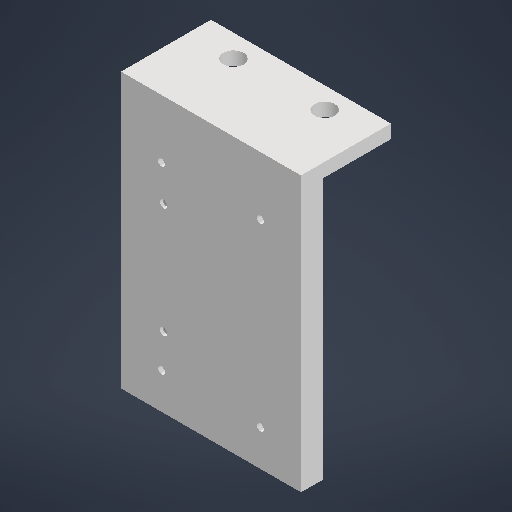
# Autodesk Inventor part: Support
Saved by Autodesk Inventor 2026.2 (Build 302298000, 298)
## iProperties
Created: 2025-11-07
Part Number: Support
Material: 일반
Document SubType Name: Modeling
Designer: alexi
Density: 1 g/cm^3
Appearance: 기본값
Author: alexi
Autodesk Inventor part; units mm, degrees
ref_plane "YZ Plane" through (0, 0, 0) normal (1, 0, 0) x (0, 1, 0)
ref_plane "XZ Plane" through (0, 0, 0) normal (0, 1, 0) x (-1, 0, 0)
ref_plane "XY Plane" through (0, 0, 0) normal (0, 0, 1) x (1, 0, 0)
ref_plane "작업 평면1" through (0, 0, 0) normal (0, 0, 1) x (1, 0, 0)
sketch "스케치1" plane through (0, 0, 0) normal (0, 0, 1) x (1, 0, 0)
  line L0 (15, -23) -> (15, 23) construction
  line L1 (15, 23) -> (-15, 23) construction
  line L2 (-15, 23) -> (-15, -23) construction
  line L3 (-15, -23) -> (15, -23) construction
  circle A0 centre (11, -20) radius 1.2 construction
  circle A1 centre (11, 20) radius 1.2 construction
  circle A2 centre (-11, -20) radius 1.2 construction
  circle A3 centre (-11, 20) radius 1.2 construction
  line L4 (20, 33) -> (-20, 33)
  line L5 (-20, 33) -> (-20, -28)
  line L6 (-20, -28) -> (20, -28)
  line L7 (20, -28) -> (20, 33)
  line L8 (-20, 30) -> (20, 30)
  line L9 (-15.525, 9.775) -> (15.475, 9.775)
  line L10 (15.475, 9.775) -> (15.475, -9.775)
  line L11 (15.475, -9.775) -> (-15.525, -9.775)
  line L12 (-15.525, -9.775) -> (-15.525, 9.775)
  circle A4 centre (-10.525, 12.275) radius 1.4
  circle A5 centre (-10.525, -12.275) radius 1.4
  point P0 (0, 0)
  dimension "d0" = 5
  dimension "d1" = 5
  dimension "d2" = 5
  dimension "d3" = 10
  dimension "d4" = 3
  dimension "d5" = 5
  dimension "d6" = 26
  dimension "d39" = 2.5
  dimension "d40" = 2.5
  constraints: 26 end point, 6 centre point, 4 horizontal, 4 parallel, 3 perpendicular, 2 point on line, 2 vertical, 17 other
  measures "d0" distance between parallel lines of L5 L2
  measures "d1" distance between parallel lines of L7 L0
  measures "d2" distance between parallel lines of L6 L3
  measures "d3" distance between parallel lines of L4 L1
  measures "d4" distance between parallel lines of L4 L8
  measures "d5" distance from line of L12 A4.centre
  measures "d6" distance from line of L10 A4.centre
  measures "d39" distance from line of L9 A4.centre
  measures "d40" distance from line of L11 A5.centre
extrude "돌출1" add sketch "스케치1" along normal blind 5 contours L7 L8 L5 L4 | L7 L6 L5 L8 | L9 L10 L11 L12 | A4 | A5
sketch "스케치2" plane through (0, 0, 0) normal (0, 0, -1) x (-1, 0, 0)
  line L0 (-15.475, 9.775) -> (-15.475, -9.775) projected
  line L1 (15.525, 9.775) -> (-15.475, 9.775) projected
  line L2 (-15.475, -9.775) -> (15.525, -9.775) projected
  line L3 (15.525, -9.775) -> (15.525, 9.775) projected
  line L4 (20, 30) -> (-20, 30) projected
  line L5 (-20, -28) -> (-20, 33) projected
  line L6 (-20, 33) -> (20, 33) projected
  line L7 (20, 33) -> (20, -28) projected
  line L8 (20, -28) -> (-20, -28) projected
  circle A0 centre (10.525, -12.275) radius 1.4
  circle A1 centre (10.525, 12.275) radius 1.4
  point P0 (0, 0)
  point P1 (-11, 20)
  point P2 (11, 20)
  point P3 (-11, -20)
  point P4 (11, -20)
  constraints: 2 centre point, 2 coincident, 8 other
extrude "돌출2" cut sketch "스케치2" against normal blind 3 contours L1 L3 L2 L0
extrude "돌출3" add sketch "스케치2" along normal blind 15 contours L4 L5 L6 L7
sketch "스케치3" plane through (-20, 33, 5) normal (0, 1, 0) x (1, 0, 0)
  line L0 (0, 0) -> (0, 20) projected
  line L1 (40, 0) -> (0, 0) projected
  line L2 (40, 20) -> (40, 0) projected
  line L3 (0, 20) -> (40, 20) projected
  line L4 (0, 0) -> (40, 20) construction
  line L5 (40, 0) -> (0, 20) construction
  point P0 (20, 5)
  point P1 (20, 10)
  point P2 (10, 15)
  point P3 (30, 15.2711)
  dimension "d15" = 20
  dimension "d16" = 5
  dimension "d17" = 10
  constraints: 4 end point, 2 midpoint
  measures "d15" horizontal distance of point (30, 15.271) point (10, 15)
  measures "d16" distance from line of L3 point (10, 15)
  measures "d17" horizontal distance of point (10, 15) point (20, 10)
hole "구멍1" at (-10, 33, -10) at (10, 33, -10.2711) direction (0, -1, 0) diameter 4.5 depth 3 tip angle 118
hole "구멍2" at (11, 20, 0) at (11, -20, 0) at (-11, -20, 0) at (-11, 20, 0) direction (0, 0, 1) diameter 1.567 depth 5 tip angle 118 thread size "M2x0.4" class "6H" standard "ANSI Metric M Profile"
hole "Hole4" at (-10.525, 12.275, 0) at (-10.525, -12.275, 0) direction (0, 0, 1) diameter 1.6942 depth 5 tip angle 118 thread size "2-56 UNC" class "2B" standard "ANSI Unified Screw Threads"
equation "\"d1\" = d0"
equation "\"d17\" = 0.5 * d15"
